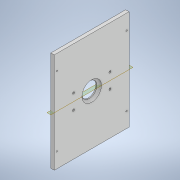
# Autodesk Inventor part: front plate
Saved by Autodesk Inventor 2020.3 (Build 243373000, 373)
## iProperties
Created: 2020-08-09
Part Number: front plate
Material: Generic
Document SubType Name: Modeling
Designer: joesp
Density: 1 g/cm^3
Appearance: Default
Author: joesp
Autodesk Inventor part; units mm, degrees
ref_plane "YZ Plane" through (0, 0, 0) normal (1, 0, 0) x (0, 1, 0)
ref_plane "XZ Plane" through (0, 0, 0) normal (0, 1, 0) x (-1, 0, 0)
ref_plane "XY Plane" through (0, 0, 0) normal (0, 0, 1) x (1, 0, 0)
sketch "Sketch1" plane through (0, 0, 0) normal (1, 0, 0) x (0, 1, 0)
  line L0 (0, 0) -> (147, 0)
  line L1 (147, 0) -> (147, 110)
  line L2 (147, 110) -> (0, 110)
  line L3 (0, 110) -> (0, 0)
  circle A0 centre (124.75, 106.25) radius 1
  circle A1 centre (124.75, 3.75) radius 1
  circle A2 centre (22.25, 3.75) radius 1
  circle A3 centre (22.25, 106.25) radius 1
  circle A4 centre (84.4635, 28.1525) radius 1.5
  circle A5 centre (84.4635, 81.8475) radius 1.5
  circle A6 centre (62.5365, 81.8475) radius 1.5
  circle A7 centre (62.5365, 28.1525) radius 1.5
  dimension "d0" = 102.5
  dimension "d1" = 102.5
  dimension "d2" = 2
  dimension "d3" = 110
  dimension "d4" = 147
  dimension "d5" = 22.25
  dimension "d6" = 22.25
  dimension "d7" = 3.75
  dimension "d8" = 3.75
  dimension "d24" = 3
  dimension "d25" = 3
  dimension "d26" = 3
  dimension "d27" = 3
  dimension "d28" = 53.695
  dimension "d29" = 21.927
  dimension "d30" = 28.1525
  dimension "d31" = 28.1525
  dimension "d32" = 62.5365
  dimension "d33" = 62.5365
  constraints: 8 centre point, 8 end point, 4 horizontal alignment, 4 vertical alignment, 3 equal radius, 2 parallel, 1 horizontal, 1 perpendicular
  measures "d0" distance of A1.centre A0.centre
  measures "d1" distance of A3.centre A0.centre
  measures "d2" diameter of A0
  measures "d3" distance of L0.end L1.end
  measures "d4" distance of L1.end L2.end
  measures "d5" distance from line of L1 A0.centre
  measures "d6" distance from line of L3 A3.centre
  measures "d7" distance from line of L2 A0.centre
  measures "d8" distance from line of L0 A1.centre
  measures "d24" diameter of A4
  measures "d25" diameter of A5
  measures "d26" diameter of A6
  measures "d27" diameter of A7
  measures "d28" distance of A5.centre A4.centre
  measures "d29" distance of A7.centre A4.centre
  measures "d30" distance from line of L2 A5.centre
  measures "d31" distance from line of L0 A4.centre
  measures "d32" distance from line of L1 A4.centre
  measures "d33" distance from line of L3 A7.centre
extrude "Extrusion1" add sketch "Sketch1" along normal blind 5
sketch "Sketch2" plane through (5, 0, 0) normal (1, 0, 0) x (0, 0, -1)
  circle A0 centre (-55, 73.5) radius 11.125
  line L0 (-110, 0) -> (0, 0) projected
  line L1 (-110, 147) -> (-110, 0) projected
  point P0 (-55, 0)
  point P1 (-110, 73.5)
  dimension "d11" = 22.25
  constraints: 2 midpoint, 1 centre point, 1 horizontal alignment, 1 vertical alignment
  measures "d11" diameter of A0
extrude "Extrusion2" cut sketch "Sketch2" against normal up to surface (5 mm away)
ref_plane "Work Plane1" through (0, 73.5, 0) normal (0, -1, 0) x (1, 0, 0)
sketch "Sketch3" plane through (0, 73.5, 0) normal (0, -1, 0) x (1, 0, 0)
  line L0 (5, 66.125) -> (5, 43.875) projected
  line L1 (0, 55) -> (5, 55) construction
  line L2 (0, 43.875) -> (0, 66.125) projected
  circle A0 centre (4, 67.125) radius 2.5
  point P0 (0, 0)
  dimension "d17" = 5
  dimension "d22" = 1
  dimension "d23" = 1
  constraints: 2 end point, 2 midpoint, 1 centre point, 1 horizontal
  measures "d17" diameter of A0
  measures "d22" horizontal distance of L0.start A0.centre
  measures "d23" horizontal distance of L0.start A0.centre
revolve "Revolution1" cut sketch "Sketch3" angle 360 about axis through (0, 73.5, 55) along (1, 0, 0)
equation "\"d1\" = d0"
equation "\"d5\" = d6"
equation "\"d7\" = d8"
equation "\"d30\" = d31"
equation "\"d32\" = d33"
body "Solid1"
